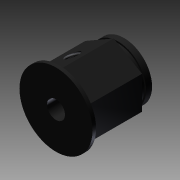
# Autodesk Inventor part: T80H-SM61
Saved by Autodesk Inventor 2012 (Build 160160000, 160)
## iProperties
Created: 2013-07-13
Part Number: T80H-SM61
Material: Default
Document SubType Name: Modeling
Designer: joe_000
Density: 1 g/cm^3
Author: joe_000
Autodesk Inventor part; units mm, degrees
ref_plane "YZ Plane" through (0, 0, 0) normal (1, 0, 0) x (0, 1, 0)
ref_plane "XZ Plane" through (0, 0, 0) normal (0, 1, 0) x (-1, 0, 0)
ref_plane "XY Plane" through (0, 0, 0) normal (0, 0, 1) x (1, 0, 0)
sketch "Sketch1" plane through (0, 0, 0) normal (0, 0, 1) x (1, 0, 0)
  line L0 (-9.4869, 5.4773) -> (0, 10.9545)
  line L1 (0, 10.9545) -> (9.4869, 5.4773)
  line L2 (9.4869, 5.4773) -> (9.4869, -5.4773)
  line L3 (9.4869, -5.4773) -> (0, -10.9545)
  line L4 (0, -10.9545) -> (-9.4869, -5.4773)
  line L5 (-9.4869, -5.4773) -> (-9.4869, 5.4773)
  point P0 (0, 0)
  point P1 (0, 0)
  dimension "d0" = 18.9738
  constraints: 12 end point, 1 coincident, 1 vertical, 13 other
  measures "d0" distance between parallel lines of L2 L5
extrude "Extrusion1" add sketch "Sketch1" along normal blind 18.034
sketch "Sketch2" plane through (0, 0, 18.034) normal (0, 0, 1) x (1, 0, 0)
  circle A0 centre (0, 0) radius 12.1793
  dimension "d3" = 24.3586
  constraints: 1 centre point, 1 coincident
  measures "d3" diameter of A0
extrude "Extrusion2" add sketch "Sketch2" along normal blind 1.2065
sketch "Sketch3" plane through (0, 0, 0) normal (0, 0, -1) x (-1, 0, 0)
  circle A0 centre (0, 0) radius 8.8455
  dimension "d6" = 17.6911
  constraints: 1 centre point, 1 coincident
  measures "d6" diameter of A0
extrude "Extrusion3" add sketch "Sketch3" along normal blind 1.4478
sketch "Sketch4" plane through (0, 0, -1.4478) normal (0, 0, -1) x (-1, 0, 0)
  circle A0 centre (0, 0) radius 9.3663
  dimension "d9" = 18.7325
  constraints: 1 centre point, 1 coincident
  measures "d9" diameter of A0
extrude "Extrusion4" add sketch "Sketch4" along normal blind 1.9939
sketch "Sketch5" plane through (0, 0, 19.2405) normal (0, 0, 1) x (1, 0, 0)
  circle A0 centre (0, 0) radius 3
  dimension "d12" = 6
  constraints: 1 centre point
  measures "d12" diameter of A0
extrude "Extrusion5" cut sketch "Sketch5" against normal through all
sketch "Sketch6" plane through (0, 10.9545, 18.034) normal (-0.5, 0.8660254, 0) x (0.8660254, 0.5, 0)
  line L0 (-10.9545, 0) -> (0, 0) projected
  line L1 (-10.9545, 18.034) -> (0, 18.034) projected
  circle A0 centre (-5.4773, 8.9662) radius 1.6336
  line L2 (-5.4773, 18.034) -> (-5.4773, 0)
  dimension "d16" = 9.0678
  constraints: 2 end point, 1 centre point, 1 midpoint, 1 point on line
  measures "d16" distance from line of L1 A0.centre
hole "Hole1" at (-4.7434, 8.2159, 9.0678) direction (0.5, -0.8660254, 0) diameter 4.6355 depth 8.89
thread "Thread1" size "10-24 UNC" class "2B" standard "ANSI Unified Screw Threads" full length
body "Solid1"
